Autodesk Fusion 360 part; units mm, degrees
(part 5 of 6)
extrude "Extrude1" add sketch "Back Panel Support Left " along normal blind 21
equation "d1 = 323 mm - 21 mm - 32 mm"

design "9V Battery Compartment"
Autodesk Fusion 360 part; units mm, degrees
sketch "Battery Body" plane through (0, 0, 0) normal (0, 0, 1) x (1, 0, 0)
  line L0 (0, 0) -> (24, 0)
  line L1 (24, 0) -> (24, 16)
  line L2 (24, 16) -> (0, 16)
  line L3 (0, 16) -> (0, 0)
  dimension "d1" = 24
  dimension "d2" = 16
  constraint horizontal L0
  constraint vertical L1
  constraint horizontal L2
  constraint vertical L3
  constraint coincident L0.start L3.end
  measures "d1" distance of L0.start L0.end
  measures "d2" distance of L0.end L1.end
extrude "Extrude1" add sketch "Battery Body" along normal blind 26 makes body 1
extrude "Extrude2" add 1 faces at (8, 10.6667, 26) along direction (0, 0, 1) blind 3 separate body on bodies 1 makes body 2
extrude "Extrude3" add 1 faces at (8, 10.6667, 29) along direction (0, 0, 1) blind 0.5 separate body on bodies 2 makes body 3
extrude "Extrude4" add 1 faces at (8, 10.6667, 29.5) along direction (0, 0, 1) blind 13.5 separate body on bodies 3 makes body 4
fillet "Fillet1" radius 1 16 edges at (0, 0, 13) (24, 0, 13) (24, 16, 13) (0, 16, 13) (0, 0, 27.5) (24, 0, 27.5) (24, 16, 27.5) (0, 16, 27.5) (0, 0, 29.25) (24, 0, 29.25) (24, 16, 29.25) (0, 16, 29.25) (0, 0, 36.25) (24, 0, 36.25) (24, 16, 36.25) (0, 16, 36.25) on bodies 1 2 3 4
sketch "Battery Terminals" plane through (0, 0, 43) normal (0, 0, 1) x (-1, 0, 0)
  arc A0 (-1, -16) -> (0, -15) centre (-1, -15) ccw
  line L0 (0, -15) -> (0, -1)
  arc A1 (0, -1) -> (-1, 0) centre (-1, -1) ccw
  line L1 (-1, 0) -> (-23, 0)
  arc A2 (-23, 0) -> (-24, -1) centre (-23, -1) ccw
  line L2 (-24, -1) -> (-24, -15)
  arc A3 (-24, -15) -> (-23, -16) centre (-23, -15) ccw
  line L3 (-23, -16) -> (-1, -16)
  circle A4 centre (-6, -8) radius 3
  circle A5 centre (-18, -8) radius 2
  circle A6 centre (-18, -8) radius 3
  circle A7 centre (-6, -8) radius 4
  dimension "d13" = 4
  dimension "d14" = 6
  dimension "d15" = 6
  dimension "d16" = 8
  dimension "d17" = 8
  dimension "d18" = 8
  dimension "d19" = 6
  dimension "d20" = 6
  constraint concentric A5 A6
  constraint concentric A4 A7
  measures "d13" diameter of A5
  measures "d14" diameter of A6
  measures "d15" diameter of A4
  measures "d16" diameter of A7
  measures "d17" distance of L1 A5.centre
  measures "d18" distance of L1 A4.centre
  measures "d19" distance of L0 A4.centre
  measures "d20" distance of L2 A5.centre
extrude "Extrude5" add sketch "Battery Terminals" along normal blind 4 separate body contours A6 | A7 makes body 5 at (15.0149, 8.2987, 44.3333) makes body 6 at (2.0199, 8.3983, 44.3333)
sketch "Battery Compartment" plane through (0, 0, 0) normal (0, 1, 0) x (1, 0, 0)
  line L0 (40, 0) -> (70, 0)
  line L1 (70, 0) -> (70, -53)
  line L2 (70, -53) -> (40, -53)
  line L3 (40, -53) -> (40, 0)
  dimension "d25" = 30
  dimension "d26" = 53
  constraint horizontal L0
  constraint vertical L1
  constraint horizontal L2
  constraint vertical L3
  measures "d25" distance of L0.start L0.end
  measures "d26" distance of L0.end L1.end
extrude "Extrude1'" add sketch "Battery Compartment" against normal blind 2 separate body makes body 7 in component "9V Battey Compartment"
sketch "Battery Compartment Fins" plane through (0, -2, 0) normal (0, -1, 0) x (1, 0, 0)
  line L0 (70, 53) -> (40, 53)
  line L1 (40, 53) -> (40, 0)
  line L2 (40, 0) -> (70, 0)
  line L3 (70, 0) -> (70, 53)
  line L4 (40, 53) -> (41, 53)
  line L5 (41, 53) -> (41, 24)
  line L6 (41, 24) -> (40, 24)
  line L7 (40, 24) -> (40, 53)
  line L8 (41, 53) -> (70, 53)
  line L9 (70, 53) -> (70, 52)
  line L10 (70, 52) -> (41, 52)
  line L11 (41, 52) -> (41, 53)
  line L12 (70, 52) -> (69, 52)
  line L13 (69, 52) -> (69, 24)
  line L14 (69, 24) -> (70, 24)
  line L15 (70, 24) -> (70, 52)
  line L16 (45, 0) -> (65, 0)
  line L17 (65, 0) -> (65, 3)
  line L18 (65, 3) -> (45, 3)
  line L19 (45, 3) -> (45, 0)
  dimension "d29" = 1
  dimension "d30" = 1
  dimension "d31" = 1
  dimension "d32" = 28
  dimension "d33" = 3
  dimension "d34" = 20
  dimension "d35" = 5
  constraint horizontal L4
  constraint vertical L5
  constraint horizontal L6
  constraint vertical L7
  constraint coincident L0.end L1.start
  constraint horizontal L8
  constraint vertical L9
  constraint horizontal L10
  constraint vertical L11
  constraint coincident L3 L9.end
  constraint horizontal L12
  constraint vertical L13
  constraint horizontal L14
  constraint vertical L15
  constraint collinear L6 L14
  constraint horizontal L16
  constraint vertical L17
  constraint horizontal L18
  constraint vertical L19
  constraint coincident L2 L16.start
  measures "d29" distance of L5.end L6.end
  measures "d30" distance of L13 L15
  measures "d31" distance of L8 L10
  measures "d32" distance of L9.end L14.end
  measures "d33" distance of L16.end L17.end
  measures "d34" distance of L16.start L16.end
  measures "d35" distance of L1 L19
extrude "Extrude2'" add sketch "Battery Compartment Fins" along normal blind 16 contours L0 L3 L5 L8 L9 L10 L11 L12 | L0 L1 L4 L5 L6 L7 L11 | L3 L10 L12 L13 L14 L15 bodies 7 in component "9V Battey Compartment"
chamfer "Chamfer1" distance 28 distance2 16 2 edges at (69.5, -18, 24) (40.5, -18, 24) measured on face at (50.3333, -18, 52.6667) measured on face at (50.3333, -18, 52.6667) on bodies 7 in component "9V Battey Compartment"
extrude "Extrude3'" add sketch "Battery Compartment Fins" along normal blind 11 contours L2 L16 L17 L18 L19 bodies 7 in component "9V Battey Compartment"
chamfer "Chamfer2" distance 2 distance2 11 1 edges at (55, -13, 0) measured on face at (58.3333, -13, 1) on bodies 7 in component "9V Battey Compartment"
sketch "Compartment Terminals" plane through (0, 0, 52) normal (0, 0, -1) x (1, 0, 0)
  line L0 (41, 2) -> (69, 2)
  line L1 (69, 2) -> (69, 18)
  line L2 (69, 18) -> (41, 18)
  line L3 (41, 18) -> (41, 2)
  circle A0 centre (49, 10) radius 3
  circle A1 centre (61, 10) radius 4
  circle A2 centre (61, 10) radius 3
  circle A3 centre (49, 10) radius 2
  line L4 (70, 2) -> (41, 2)
  dimension "d44" = 12
  dimension "d45" = 6
  dimension "d46" = 8
  dimension "d47" = 4
  dimension "d48" = 6
  dimension "d49" = 8
  dimension "d51" = 8
  dimension "d52" = 8
  constraint concentric A1 A2
  constraint concentric A0 A3
  measures "d44" distance of A0.centre A1.centre
  measures "d45" diameter of A2
  measures "d46" diameter of A1
  measures "d47" diameter of A3
  measures "d48" diameter of A0
  measures "d49" distance of A0.centre L4
  measures "d51" distance of A1.centre L4
  measures "d52" distance of L3 A0.centre
extrude "Extrude6" add sketch "Compartment Terminals" along normal blind 4 separate body contours A0 | A1 makes body 8 at (51.9851, -9.7013, 50.6667) makes body 9 at (64.9801, -9.6017, 50.6667)
fillet "Fillet3" radius 0.5 4 edges at (46.203, -8.9152, 48) (47.1353, -10.7232, 48) (58.203, -11.0848, 48) (57.2707, -8.5535, 48) on bodies 8 9
copy_body "CutPasteBodies1" bodies 9 removing the originals makes body 10 in component "9V Battey Compartment"
copy_body "CutPasteBodies2" bodies 8 removing the originals makes body 11 in component "9V Battey Compartment"
copy_body "Body->Comp1" bodies 1 removing the originals makes body 12 in component "9V Battery"
copy_body "CutPasteBodies1'" bodies 2 removing the originals makes body 13 in component "9V Battery"
copy_body "CutPasteBodies2'" bodies 3 removing the originals makes body 14 in component "9V Battery"
copy_body "CutPasteBodies3" bodies 4 removing the originals makes body 15 in component "9V Battery"
copy_body "CutPasteBodies4" bodies 5 removing the originals makes body 16 in component "9V Battery"
copy_body "CutPasteBodies5" bodies 6 removing the originals makes body 17 in component "9V Battery"
fillet "Fillet1'" radius 0.5 4 edges at (20.797, 9.0848, 47) (19.8647, 7.2768, 47) (8.797, 6.9152, 47) (9.7293, 9.4465, 47) on bodies 16 17 in component "9V Battery"
sketch "Compartment Bottom Fin Round Part" plane through (25, 0, 0) normal (1, 0, 0) x (0, 1, 0)
  line L0 (-11, 2) -> (0, 0)
  line L1 (0, 0) -> (0, 3)
  line L2 (0, 3) -> (-11, 3)
  line L3 (-11, 3) -> (-11, 2)
  ellipse E0 centre (-9, 3) end of major axis (-9, 2.5) minor radius 2
  line L4 (-9, 3.5) -> (-9, 2.5) construction
  line L5 (-11, 3) -> (-7, 3) construction
  dimension "d66" = 4
  dimension "d67" = 2
  constraint coincident L2 E0.centre
  constraint perpendicular L2 L4
  constraint coincident E0 L4.start
  constraint coincident E0 L4.end
  constraint coincident E0 L2.end
  constraint coincident E0 L5.end
  measures "d67" distance of L2.end E0.centre
extrude "Extrude4'" add sketch "Compartment Bottom Fin Round Part" against normal blind 20 contours L2 E0 picked at (-9.0518, 3.1662) sketch seen with x (1, 0, 0) y (0, 1, 0) z (0, 0, 1) at (40, -2, 0) bodies 7 in component "9V Battey Compartment"
combine "Combine1" operation add target body 12 tool bodies 13 14 in component "9V Battery"
component "9V Battey Compartment" placed x (1, 0, 0) y (0, 1, 0) z (0, 0, 1) at (-40, 2, 0)
component "9V Battery" placed x (1, 0, 0) y (0, 1, 0) z (0, 0, 1) at (3, -16, 5)

design "Savöx SH 0255 MG Micro Servo"
Autodesk Fusion 360 part; units mm, degrees
sketch "Servo Side Profile" plane through (0, 0, 0) normal (1, 0, 0) x (0, 1, 0)
  line L0 (0, 0) -> (22, 0)
  line L1 (22, 0) -> (22, 16)
  line L2 (22, 16) -> (27, 16)
  line L3 (27, 16) -> (27, 18)
  line L4 (27, 18) -> (22, 18)
  line L5 (22, 18) -> (22, 22)
  line L6 (22, 22) -> (0, 22)
  line L7 (0, 22) -> (0, 18)
  line L8 (0, 18) -> (-5, 18)
  line L9 (-5, 18) -> (-5, 16)
  line L10 (-5, 16) -> (0, 16)
  line L11 (0, 16) -> (0, 0)
  dimension "d1" = 22
  dimension "d2" = 22
  dimension "d3" = 16
  dimension "d4" = 16
  dimension "d5" = 2
  dimension "d6" = 2
  dimension "d7" = 4
  dimension "d9" = 5
  dimension "d10" = 5
  constraint coincident L0.start L11.end
  constraint horizontal L0
  constraint perpendicular L0 L1
  constraint perpendicular L1 L2
  constraint perpendicular L2 L3
  constraint perpendicular L3 L4
  constraint perpendicular L4 L5
  constraint perpendicular L3 L6
  constraint perpendicular L6 L7
  constraint perpendicular L3 L8
  constraint perpendicular L8 L9
  constraint perpendicular L9 L10
  constraint perpendicular L0 L11
  constraint collinear L7 L11
  measures "d1" distance of L0.start L0.end
  measures "d2" distance of L5.end L6.end
  measures "d3" distance of L0.end L1.end
  measures "d4" distance of L10.end L0.start
  measures "d5" distance of L2.end L3.end
  measures "d6" distance of L8.end L9.end
  measures "d7" distance of L6.end L7.end
  measures "d9" distance of L3.end L4.end
  measures "d10" distance of L7.end L8.end
extrude "Extrude1" add sketch "Servo Side Profile" along normal blind 11 makes body 1
sketch "Top Cylinders" plane through (0, 0, 22) normal (0, 0, 1) x (-1, 0, 0)
  line L0 (0, -22) -> (0, 0)
  line L1 (0, 0) -> (-11, 0)
  line L2 (-11, 0) -> (-11, -22)
  line L3 (-11, -22) -> (0, -22)
  circle A0 centre (-5.5, -5.5) radius 5.5
  circle A1 centre (-5.5, -11) radius 2.5
  dimension "d13" = 5.5
  dimension "d14" = 5.5
  dimension "d15" = 11
  dimension "d16" = 5.5
  dimension "d17" = 11
  dimension "d18" = 5
  measures "d13" distance of L2 A0.centre
  measures "d14" distance of L1 A0.centre
  measures "d15" diameter of A0
  measures "d16" distance of L2 A1.centre
  measures "d17" distance of L1 A1.centre
  measures "d18" diameter of A1
extrude "Extrude2" add sketch "Top Cylinders" along normal blind 5 contours A0 A1 | A0 A1 | A0 A1 bodies 1
sketch "Turning Gear" plane through (0, 0, 27) normal (0, 0, 1) x (-1, 0, 0)
  arc A0 (-7.9346, -10.4318) -> (-3.0654, -10.4318) centre (-5.5, -11) ccw
  arc A1 (-3.0654, -10.4318) -> (-7.9346, -10.4318) centre (-5.5, -5.5) ccw
  circle A2 centre (-5.5, -5.5) radius 2.5
  dimension "d21" = 5
  constraint concentric A1 A2
  measures "d21" diameter of A2
extrude "Extrude3" add sketch "Turning Gear" along normal blind 3 separate body contours A2 makes body 2
equation "d13 = ( 11 / 2 ) * 1 mm"
equation "d14 = ( 11 / 2 ) * 1 mm"
equation "d16 = ( 11 / 2 ) * 1 mm"
equation "d17 = ( 22 / 2 ) * 1 mm"

design "Colour Detection Mechanism Top Panel Placeholder"
Autodesk Fusion 360 part; units mm, degrees
sketch "Sorting Mechanism Top Panel Placeholder" plane through (0, 0, 0) normal (0, 0, 1) x (1, 0, 0)
  line L0 (0, 0) -> (28, 0)
  line L1 (28, 0) -> (28, 10)
  line L2 (28, 10) -> (0, 10)
  line L3 (0, 10) -> (0, 0)
  dimension "d1" = 10
  dimension "d2" = 28
  constraint horizontal L0
  constraint vertical L1
  constraint horizontal L2
  constraint vertical L3
  constraint coincident L0.start L3.end
  measures "d1" distance of L0.end L1.end
  measures "d2" distance of L0.start L0.end
extrude "Extrude1" add sketch "Sorting Mechanism Top Panel Placeholder" along normal blind 12

design "Unsorted Smarties Top Panel"
Autodesk Fusion 360 part; units mm, degrees
sketch "Unsorted Smarties Top" plane through (0, 0, 0) normal (0, 0, 1) x (1, 0, 0)
  line L0 (0, 0) -> (270, 0)
  line L1 (270, 0) -> (270, 48)
  line L2 (270, 48) -> (0, 48)
  line L3 (0, 48) -> (0, 0)
  dimension "d1" = 270
  dimension "d2" = 48
  constraint horizontal L0
  constraint vertical L1
  constraint horizontal L2
  constraint vertical L3
  constraint coincident L0.start L3.end
  measures "d1" distance of L0.start L0.end
  measures "d2" distance of L0.end L1.end
extrude "Extrude1" add sketch "Unsorted Smarties Top" along normal blind 6
sketch "Sketch2" plane through (0, 0, 0) normal (0, 0, -1) x (1, 0, 0)
  line L0 (0, 0) -> (0, -48)
  line L1 (0, -48) -> (270, -48)
  line L2 (270, -48) -> (270, 0)
  line L3 (270, 0) -> (0, 0)
  line L4 (5, -10) -> (265, -10)
  line L5 (265, -10) -> (265, -20)
  line L6 (265, -20) -> (5, -20)
  line L7 (5, -20) -> (5, -10)
  line L8 (5, -29) -> (265, -29)
  line L9 (265, -29) -> (265, -39)
  line L10 (265, -39) -> (5, -39)
  line L11 (5, -39) -> (5, -29)
  dimension "d6" = 5
  dimension "d7" = 5
  dimension "d8" = 5
  dimension "d9" = 5
  dimension "d10" = 10
  dimension "d11" = 10
  dimension "d12" = 9
  dimension "d13" = 10
  constraint horizontal L4
  constraint vertical L5
  constraint horizontal L6
  constraint vertical L7
  constraint horizontal L8
  constraint vertical L9
  constraint horizontal L10
  constraint vertical L11
  measures "d6" distance of L2 L5
  measures "d7" distance of L2 L9
  measures "d8" distance of L0 L7
  measures "d9" distance of L0 L11
  measures "d10" distance of L4.start L6.end
  measures "d11" distance of L3 L4
  measures "d12" distance of L6 L8
  measures "d13" distance of L8.start L10.end
extrude "Extrude2" cut sketch "Sketch2" against normal blind 4 contours L4 L5 L6 L7 | L8 L9 L10 L11
sketch "Sketch3" plane through (0, 0, 4) normal (0, 0, -1) x (1, 0, 0)
  line L0 (5, -20) -> (265, -20)
  line L1 (265, -20) -> (265, -10)
  line L2 (265, -10) -> (5, -10)
  line L3 (5, -10) -> (5, -20)
  line L4 (265, -10) -> (255, -10)
  line L5 (255, -10) -> (255, -20)
  line L6 (255, -20) -> (265, -20)
  line L7 (265, -20) -> (265, -10)
  line L8 (265, -29) -> (255, -29)
  line L9 (255, -29) -> (255, -39)
  line L10 (255, -39) -> (265, -39)
  line L11 (265, -39) -> (265, -29)
  constraint horizontal L4
  constraint vertical L5
  constraint horizontal L6
  constraint vertical L7
  constraint coincident L0 L5.end
  constraint coincident L1.end L2.start
  constraint horizontal L8
  constraint vertical L9
  constraint horizontal L10
  constraint vertical L11
extrude "Extrude3" cut sketch "Sketch3" against normal blind 2 contours L0 L1 L2 L4 L5 L6 L7 | L8 L9 L10 L11
equation "mdfThickness = 6 mm"
equation "d4 = mdfThickness"

design "Control Panel Front"
Autodesk Fusion 360 part; units mm, degrees
sketch "Control Panel Front" plane through (0, 0, 0) normal (0, 1, 0) x (1, 0, 0)
  line L0 (0, 0) -> (270, 0)
  line L1 (270, 0) -> (270, -43)
  line L2 (270, -43) -> (0, -43)
  line L3 (0, -43) -> (0, 0)
  dimension "d6" = 270
  dimension "d7" = 43
  constraint horizontal L0
  constraint vertical L1
  constraint horizontal L2
  constraint vertical L3
  constraint coincident L0.start L3.end
  measures "d6" distance of L0.start L0.end
  measures "d7" distance of L0.end L1.end
extrude "Extrude1" add sketch "Control Panel Front" along normal blind 6
equation "MDFThickness = 6 mm"
equation "d2 = MDFThickness"
equation "d7 = sidePanelControlPanelHeight - 2 * sidePanelClearance - 2 * MDFThickness"
equation "sidePanelClearance = 10 mm"
equation "sidePanelControlPanelHeight = 75 mm"

design "Name Sign LED Holder"
Autodesk Fusion 360 part; units mm, degrees
sketch "Sketch1" plane through (0, 0, 0) normal (0, 1, 0) x (1, 0, 0)
  line L0 (2.4744, -68.9852) -> (7.4744, -68.9852)
  line L1 (7.4744, -68.9852) -> (7.4744, -22.3387)
  line L2 (7.4744, -22.3387) -> (36.754, -10.3303)
  line L3 (36.754, -10.3303) -> (34.8567, -5.7042)
  line L4 (34.8567, -5.7042) -> (2.4744, -18.9852)
  line L5 (2.4744, -18.9852) -> (2.4744, -68.9852)
  line L6 (2.4744, -68.9852) -> (7.4744, -66.9345)
  line L7 (34.8567, -5.7042) -> (34.8567, -11.1084)
  dimension "d1" = 5
  dimension "d2" = 5
  dimension "d3" = 112.3
  dimension "d16" = 50
  dimension "d18" = 22.3
  dimension "d20" = 35
  constraint horizontal L0
  constraint perpendicular L0 L1
  constraint perpendicular L2 L3
  constraint perpendicular L0 L5
  constraint parallel L2 L4
  constraint coincident L1 L6.end
  constraint parallel L2 L6
  constraint coincident L2 L7.end
  constraint vertical L7
  measures "d1" distance of L0.start L0.end
  measures "d2" distance of L2.end L3.end
  measures "d3" angle of L1 L2
  measures "d16" distance of L0.start L4.end
  measures "d18" angle of L0 L6
  measures "d20" distance of L3.end L4.end
extrude "Extrude1" add sketch "Sketch1" along normal blind 220 contours L1 L2 L4 L5 L6 L7
sketch "Sketch2" plane through (2.4744, 0, 0) normal (-1, 0, 0) x (0, -1, 0)
  line L0 (0, 18.9852) -> (0, 68.9852)
  line L1 (-220, 68.9852) -> (-220, 18.9852)
  line L2 (-220, 18.9852) -> (0, 18.9852)
  line L3 (-215, 66.9852) -> (-5, 66.9852)
  line L4 (-5, 66.9852) -> (-5, 56.9852)
  line L5 (-5, 56.9852) -> (-215, 56.9852)
  line L6 (-215, 56.9852) -> (-215, 66.9852)
  line L7 (-215, 52.9852) -> (-5, 52.9852)
  line L8 (-5, 52.9852) -> (-5, 42.9852)
  line L9 (-5, 42.9852) -> (-215, 42.9852)
  line L10 (-215, 42.9852) -> (-215, 52.9852)
  line L11 (-5, 66.9852) -> (-15, 66.9852)
  line L12 (-15, 56.9852) -> (-5, 56.9852)
  line L13 (-5, 56.9852) -> (-5, 66.9852)
  line L14 (-5, 52.9852) -> (-15, 52.9852)
  line L15 (-15, 42.9852) -> (-5, 42.9852)
  line L16 (-5, 42.9852) -> (-5, 52.9852)
  line L17 (0, 68.9852) -> (-220, 68.9852)
  dimension "d6" = 210
  dimension "d7" = 210
  dimension "d8" = 5
  dimension "d9" = 5
  dimension "d12" = 10
  dimension "d13" = 10
  dimension "d22" = 4
  dimension "d30" = 2
  constraint horizontal L3
  constraint vertical L4
  constraint horizontal L5
  constraint vertical L6
  constraint horizontal L7
  constraint vertical L8
  constraint horizontal L9
  constraint vertical L10
  constraint horizontal L11
  constraint horizontal L12
  constraint vertical L13
  constraint coincident L5 L12.start
  constraint horizontal L14
  constraint horizontal L15
  constraint vertical L16
  constraint coincident L9 L15.start
  measures "d6" distance of L3.start L3.end
  measures "d7" distance of L8.end L9.end
  measures "d8" distance of L1 L6
  measures "d9" distance of L0 L8
  measures "d12" distance of L3.start L5.end
  measures "d13" distance of L7.start L9.end
  measures "d22" distance of L5 L7
  measures "d30" distance of L3 L17
extrude "Extrude2" cut sketch "Sketch2" against normal blind 3 contours L3 L4 L5 L6 L11 L12 L13 | L7 L8 L9 L10 L14 L15 L16
sketch "Sketch3" plane through (5.4744, 0, 0) normal (-1, 0, 0) x (0, -1, 0)
  line L0 (-215, 56.9852) -> (-5, 56.9852)
  line L1 (-5, 56.9852) -> (-5, 66.9852)
  line L2 (-5, 66.9852) -> (-215, 66.9852)
  line L3 (-215, 66.9852) -> (-215, 56.9852)
  line L4 (-5, 66.9852) -> (-15, 66.9852)
  line L5 (-15, 66.9852) -> (-15, 56.9852)
  line L6 (-15, 56.9852) -> (-5, 56.9852)
  line L7 (-5, 56.9852) -> (-5, 66.9852)
  dimension "d33" = 10
  dimension "d34" = 10
  constraint horizontal L4
  constraint vertical L5
  constraint horizontal L6
  constraint vertical L7
  constraint coincident L0 L5.end
  constraint coincident L1.end L2.start
  measures "d33" distance of L1.end L4.end
  measures "d34" distance of L1.end L0.end
sketch "Sketch4" plane through (5.4744, 0, 0) normal (-1, 0, 0) x (0, -1, 0)
  line L0 (-215, 42.9852) -> (-5, 42.9852)
  line L1 (-5, 42.9852) -> (-5, 52.9852)
  line L2 (-215, 52.9852) -> (-215, 42.9852)
  line L3 (-5, 52.9852) -> (-15, 52.9852)
  line L4 (-15, 52.9852) -> (-15, 42.9852)
  line L5 (-15, 42.9852) -> (-5, 42.9852)
  line L6 (-5, 42.9852) -> (-5, 52.9852)
  line L7 (-5, 52.9852) -> (-215, 52.9852)
  dimension "d26" = 10
  dimension "d27" = 10
  constraint horizontal L3
  constraint vertical L4
  constraint horizontal L5
  constraint vertical L6
  constraint coincident L0 L4.end
  constraint coincident L1.end L3.start
  measures "d26" distance of L1.end L3.end
  measures "d27" distance of L1.end L0.end
extrude "Extrude3" cut sketch "Sketch3" sketch "Sketch4" against normal blind 2 contours L0 L1 L2 L4 L5 L6 L7 of sketch 2 contours L0 L1 L3 L4 L5 L6 L7
equation "d4 = 200 mm + 10 mm + 5 mm + 5 mm"
equation "d6 = 200 mm + 10 mm"
equation "d7 = 200 mm + 10 mm"

design "Smartie Hopper"
Autodesk Fusion 360 part; units mm, degrees
sketch "Bottom opening" plane through (0, 0, 0) normal (0, 0, 1) x (1, 0, 0)
  line L0 (0, 0) -> (18, 0)
  line L1 (18, 0) -> (18, 18)
  line L2 (18, 18) -> (0, 18)
  line L3 (0, 18) -> (0, 0)
  line L4 (-4, 22) -> (22, 22)
  line L5 (22, 22) -> (22, -4)
  line L6 (22, -4) -> (-4, -4)
  line L7 (-4, -4) -> (-4, 22)
  dimension "d3" = 18
  dimension "d4" = 18
  dimension "d5" = 4
  dimension "d6" = 4
  dimension "d7" = 4
  dimension "d8" = 4
  constraint horizontal L0
  constraint vertical L1
  constraint horizontal L2
  constraint vertical L3
  constraint coincident L0.start L3.end
  constraint horizontal L4
  constraint vertical L5
  constraint horizontal L6
  constraint vertical L7
  measures "d3" distance of L0.start L0.end
  measures "d4" distance of L0.end L1.end
  measures "d5" distance of L2 L4
  measures "d6" distance of L0 L6
  measures "d7" distance of L1 L5
  measures "d8" distance of L3 L7
ref_plane "WorkPlane1" through (0, 0, 34) normal (0, 0, 1) x (1, 0, 0)
sketch "Top opening" plane through (0, 0, 34) normal (0, 0, 1) x (1, 0, 0)
  line L0 (18, 18) -> (0, 18)
  line L1 (18, 0) -> (18, 18)
  line L2 (0, 0) -> (18, 0)
  line L3 (0, 18) -> (0, 0)
  line L4 (-4, 22) -> (22, 22)
  line L5 (22, -4) -> (-4, -4)
  line L6 (22, 22) -> (22, -4)
  line L7 (-4, -4) -> (-4, 22)
  line L8 (-36, 44) -> (54, 44)
  line L9 (54, 44) -> (54, -26)
  line L10 (54, -26) -> (-36, -26)
  line L11 (-36, -26) -> (-36, 44)
  line L12 (-39, 47) -> (57, 47)
  line L13 (57, 47) -> (57, -29)
  line L14 (57, -29) -> (-39, -29)
  line L15 (-39, -29) -> (-39, 47)
  line L16 (-40, 48) -> (58, 48)
  line L17 (58, 48) -> (58, -30)
  line L18 (58, -30) -> (-40, -30)
  line L19 (-40, -30) -> (-40, 48)
  dimension "d14" = 3
  dimension "d15" = 4
  dimension "d16" = 3
  dimension "d17" = 4
  dimension "d18" = 90
  dimension "d19" = 70
  dimension "d20" = 3
  dimension "d21" = 4
  dimension "d22" = 3
  dimension "d23" = 4
  dimension "d24" = 32
  dimension "d25" = 32
  dimension "d26" = 22
  dimension "d27" = 22
  constraint horizontal L8
  constraint vertical L9
  constraint horizontal L10
  constraint vertical L11
  constraint horizontal L12
  constraint vertical L13
  constraint horizontal L14
  constraint vertical L15
  constraint horizontal L16
  constraint vertical L17
  constraint horizontal L18
  constraint vertical L19
  measures "d14" distance of L9 L13
  measures "d15" distance of L9 L17
  measures "d16" distance of L11 L15
  measures "d17" distance of L11 L19
  measures "d18" distance of L8.start L8.end
  measures "d19" distance of L8.end L9.end
  measures "d20" distance of L8 L12
  measures "d21" distance of L8 L16
  measures "d22" distance of L10 L14
  measures "d23" distance of L10 L18
  measures "d24" distance of L7 L11
  measures "d25" distance of L6 L9
  measures "d26" distance of L4 L8
  measures "d27" distance of L5 L10
loft "Loft1" add profiles "Top opening", "Bottom opening" section 1 contours L8 L9 L10 L11 | L12 L13 L14 L15 | L16 L17 L18 L19 section 2 contours L0 L1 L2 L3 | L4 L5 L6 L7
extrude "Extrude1" cut sketch "Top opening" against normal blind 6 contours L16 L17 L18 L19
extrude "Extrude4" add 1 faces at (25, -3.6667, 34) along direction (0, 0, -1) blind 6
sketch "Support lip" plane through (57, 0, 0) normal (1, 0, 0) x (0, 1, 0)
  line L0 (47, 28) -> (47, 34)
  line L1 (47, 34) -> (-29, 34)
  line L2 (-29, 34) -> (-29, 28)
  line L3 (-29, 28) -> (77, 28)
  line L4 (77, 28) -> (77, 23)
  line L5 (77, 23) -> (-29, 23)
  line L6 (-29, 23) -> (-29, 28)
  line L7 (-29, 28) -> (47, 28)
  line L8 (-29, 28) -> (9, 28)
  line L9 (9, 28) -> (9, 23)
  line L10 (9, 23) -> (-29, 23)
  line L11 (-29, 23) -> (-29, 28)
  dimension "d31" = 6
  dimension "d34" = 5
  dimension "d35" = 30
  dimension "d50" = 38
  constraint horizontal L3
  constraint vertical L4
  constraint horizontal L5
  constraint vertical L6
  constraint collinear L2 L6
  constraint horizontal L8
  constraint vertical L9
  constraint horizontal L10
  constraint vertical L11
  constraint coincident L5 L9.end
  constraint coincident L2.end L3.start
  measures "d31" distance of L1 L3
  measures "d34" distance of L2.end L5.end
  measures "d35" distance of L0.end L3.end
  measures "d50" distance of L9 L11
extrude "Extrude2" add sketch "Support lip" along normal blind 30 and the other way blind 126 contours L3 L5 L6 L7 L8 L9 L10 L11
extrude "Extrude5" add sketch "Support lip" against normal blind 78 from surface at -48 contours L3 L4 L5 L7 L9
fillet "Fillet4" radius 5 5 edges at (87, 9, 25.5) (87, -29, 25.5) (9, 77, 25.5) (-69, 77, 25.5) (-69, -29, 25.5)
loft "Loft2" cut profiles "Top opening", "Bottom opening" section 1 contours L8 L9 L10 L11 section 2 contours L0 L1 L2 L3
fillet "Fillet3" radius 12.803 4 edges at (-18, 31, 17) (-18, -13, 17) (36, -13, 17) (36, 31, 17)
fillet "Fillet5" radius 18.495 4 edges at (-16.1765, -12.7941, 11.5) (-16.1765, 30.7941, 11.5) (36.8235, 32.7059, 14) (34.1765, -12.7941, 11.5)
equation "bottom_outlet_size = 18 mm"
equation "hopper_wall_thickness = 4 mm"
equation "d3 = bottom_outlet_size"
equation "d4 = bottom_outlet_size"
equation "d5 = hopper_wall_thickness"
equation "d6 = hopper_wall_thickness"
equation "d7 = hopper_wall_thickness"
equation "d8 = hopper_wall_thickness"
equation "hopper_height = 34 mm"
equation "d10 = hopper_height"
equation "acrylic_thickness = 3 mm"
equation "top_outlet_width = 90 mm"
equation "top_outlet_depth = 70 mm"
equation "d14 = acrylic_thickness"
equation "d15 = hopper_wall_thickness"
equation "d16 = acrylic_thickness"
equation "d17 = hopper_wall_thickness"
equation "d18 = top_outlet_width"
equation "d19 = top_outlet_depth"
equation "d20 = acrylic_thickness"
equation "d21 = hopper_wall_thickness"
equation "d22 = acrylic_thickness"
equation "d23 = hopper_wall_thickness"
equation "d24 = ( top_outlet_width - ( bottom_outlet_size + 2 * hopper_wall_thickness ) ) / 2"
equation "d26 = ( top_outlet_depth - ( bottom_outlet_size + 2 * hopper_wall_thickness ) ) / 2"
equation "MDF_thickness = 6 mm"
equation "d31 = MDF_thickness"
equation "support_lip_width = 30 mm"
equation "support_lip_thickness = 5 mm"
equation "d34 = support_lip_thickness"
equation "d35 = support_lip_width"
equation "d36 = support_lip_width"
equation "d38 = ( top_outlet_width + 2 * acrylic_thickness ) + support_lip_width"
equation "d50 = ( top_outlet_depth / 2 ) + acrylic_thickness"
equation "d51 = -( top_outlet_width / 2 ) - acrylic_thickness"
equation "d52 = -( top_outlet_width / 2 ) - acrylic_thickness - support_lip_width"

design "1.5 Volt Label"
Autodesk Fusion 360 part; units mm, degrees
sketch "Sticker" plane through (0, 0, 0) normal (0, 1, 0) x (1, 0, 0)
  line L0 (0, 0) -> (35, 0)
  line L1 (35, 0) -> (35, -12)
  line L2 (35, -12) -> (0, -12)
  line L3 (0, -12) -> (0, 0)
  dimension "d1" = 35
  dimension "d2" = 12
  constraint horizontal L0
  constraint vertical L1
  constraint horizontal L2
  constraint vertical L3
  constraint coincident L0.start L3.end
  measures "d1" distance of L0.start L0.end
  measures "d2" distance of L0.end L1.end
extrude "Extrude1" add sketch "Sticker" along normal blind 0.01 makes body 1
sketch "Text" plane through (0, 0, 0) normal (0, -1, 0) x (1, 0, 0)
  line L0 (35, 12) -> (0, 12)
  line L1 (0, 12) -> (0, 0)
  line L2 (0, 0) -> (35, 0)
  line L3 (35, 0) -> (35, 12)
  line L4 (0, 0) -> (35, 0) construction
  line L5 (35, 0) -> (35, 12) construction
  line L6 (35, 12) -> (0, 12) construction
  line L7 (0, 12) -> (0, 0) construction
  dimension "d5" = 5
  text T0 "2 × 1.5 V" font "Arial" height 5 align centre middle in box 35 x 12 at (0, 0) x (1, 0) y (0, 1) spacing 1 kerned
  constraint coincident L2.end
  constraint coincident L0.end
extrude "Extrude2" add sketch "Text" along normal blind 0.01 separate body text T0 makes body 2 at (10.575, 0, 6.465) makes body 3 at (27.7817, 0, 7.2892) makes body 4 at (22.8908, 0, 8.2362) makes body 5 at (20.1748, 0, 3.7331) makes body 6 at (17.5872, 0, 6.4775) makes body 7 at (4.9417, 0, 3.6967)

design "Base Plate Support"
Autodesk Fusion 360 part; units mm, degrees
sketch "Control Panel Support" plane through (0, 0, 0) normal (1, 0, 0) x (0, 1, 0)
  line L0 (0, 0) -> (48, 0)
  line L1 (48, 0) -> (48, 50)
  line L2 (48, 50) -> (0, 50)
  line L3 (0, 50) -> (0, 0)
  dimension "d1" = 48
  dimension "d2" = 50
  constraint horizontal L0
  constraint vertical L1
  constraint horizontal L2
  constraint vertical L3
  constraint coincident L0.start L3.end
  measures "d1" distance of L0.start L0.end
  measures "d2" distance of L0.end L1.end
extrude "Extrude1" add sketch "Control Panel Support" along normal blind 12
equation "pineThickness = 12 mm"
equation "d4 = pineThickness"
equation "mdfThickness = 6 mm"

design "Back Panel"
Autodesk Fusion 360 part; units mm, degrees
sketch "Back Panel" plane through (0, 0, 0) normal (1, 0, 0) x (0, 1, 0)
  line L0 (0, 0) -> (6, 0)
  line L1 (6, 0) -> (6, 500.8)
  line L2 (0, 500.8) -> (0, 0)
  line L3 (0, 500.8) -> (0, 503.263)
  line L4 (6, 500.8) -> (0, 503.263)
  dimension "d8" = 6
  dimension "d9" = 500.8
  dimension "d10" = 2.463
  dimension "d11" = 112.318
  constraint horizontal L0
  constraint vertical L1
  constraint vertical L2
  constraint coincident L0.start L2.end
  measures "d8" distance of L0.start L0.end
  measures "d9" distance of L0.end L1.end
  measures "d10" distance of L2.start L3.end
  measures "d11" angle of L1 L4
extrude "Extrude2" add sketch "Back Panel" along normal blind 270
sketch "Switch Hole" plane through (0, 6, 0) normal (0, 1, 0) x (-1, 0, 0)
  line L0 (0, 0) -> (0, 500.8)
  line L1 (0, 500.8) -> (-270, 500.8)
  line L2 (-270, 500.8) -> (-270, 0)
  line L3 (-270, 0) -> (0, 0)
  line L4 (-234, 37) -> (-215, 37)
  line L5 (-215, 37) -> (-215, 24)
  line L6 (-215, 24) -> (-234, 24)
  line L7 (-234, 24) -> (-234, 37)
  dimension "d14" = 19
  dimension "d15" = 13
  dimension "d16" = 36
  dimension "d17" = 24
  constraint horizontal L4
  constraint vertical L5
  constraint horizontal L6
  constraint vertical L7
  measures "d14" distance of L5.end L6.end
  measures "d15" distance of L4.end L5.end
  measures "d16" distance of L2 L7
  measures "d17" distance of L3 L6
extrude "Extrude3" cut sketch "Switch Hole" against normal blind 6 contours L4 L5 L6 L7
sketch "Bottom Access Panel" plane through (0, 6, 0) normal (0, 1, 0) x (-1, 0, 0)
  line L0 (-215, 37) -> (-215, 24)
  line L1 (-215, 24) -> (-234, 24)
  line L2 (-234, 24) -> (-234, 37)
  line L3 (-234, 37) -> (-215, 37)
  line L4 (0, 0) -> (0, 500.8)
  line L5 (0, 500.8) -> (-270, 500.8)
  line L6 (-270, 500.8) -> (-270, 0)
  line L7 (-270, 0) -> (0, 0)
  line L8 (-205, 188) -> (-65, 188)
  line L9 (-65, 188) -> (-65, 48)
  line L10 (-65, 48) -> (-205, 48)
  line L11 (-205, 48) -> (-205, 188)
  dimension "d20" = 48
  dimension "d21" = 65
  dimension "d22" = 65
  dimension "d28" = 140
  dimension "d29" = 140
  dimension "d30" = 24
  dimension "d31" = 11
  dimension "d32" = 13
  dimension "d33" = 188
  constraint horizontal L8
  constraint vertical L9
  constraint horizontal L10
  constraint vertical L11
  measures "d20" distance of L7 L10
  measures "d21" distance of L6 L11
  measures "d22" distance of L4 L9
  measures "d28" distance of L8.end L9.end
  measures "d29" distance of L9.end L10.end
  measures "d30" distance of L1 L7
  measures "d31" distance of L3 L10
  measures "d32" distance of L1 L3
  measures "d33" distance of L7 L8
extrude "Extrude4" cut sketch "Bottom Access Panel" against normal blind 6 contours L8 L9 L10 L11
fillet "Fillet1" radius 8 4 edges at (65, 3, 188) (65, 3, 48) (205, 3, 48) (205, 3, 188)
sketch "Top Access Panel" plane through (0, 6, 0) normal (0, 1, 0) x (-1, 0, 0)
  line L0 (-65, 180) -> (-65, 56)
  arc A0 (-73, 48) -> (-65, 56) centre (-73, 56) ccw
  line L1 (-73, 48) -> (-197, 48)
  arc A1 (-205, 56) -> (-197, 48) centre (-197, 56) ccw
  line L2 (-205, 56) -> (-205, 180)
  arc A2 (-197, 188) -> (-205, 180) centre (-197, 180) ccw
  line L3 (-197, 188) -> (-73, 188)
  arc A3 (-65, 180) -> (-73, 188) centre (-73, 180) ccw
  line L4 (-215, 37) -> (-215, 24)
  line L5 (-215, 24) -> (-234, 24)
  line L6 (-234, 24) -> (-234, 37)
  line L7 (-234, 37) -> (-215, 37)
  line L8 (0, 0) -> (0, 500.8)
  line L9 (0, 500.8) -> (-270, 500.8)
  line L10 (-270, 500.8) -> (-270, 0)
  line L11 (-270, 0) -> (0, 0)
  line L12 (-195, 473.263) -> (-75, 473.263)
  line L13 (-75, 473.263) -> (-75, 383.263)
  line L14 (-75, 383.263) -> (-195, 383.263)
  line L15 (-195, 383.263) -> (-195, 473.263)
  line L16 (-180, 473.263) -> (-90, 473.263)
  line L17 (0, 503.263) -> (-270, 503.263)
  dimension "d34" = 120
  dimension "d35" = 140
  dimension "d36" = 75
  dimension "d37" = 75
  dimension "d38" = 65
  dimension "d39" = 65
  dimension "d45" = 90
  dimension "d49" = 30
  constraint horizontal L12
  constraint vertical L13
  constraint horizontal L14
  constraint vertical L15
  constraint coincident L12 L16.start
  measures "d34" distance of L13.end L14.end
  measures "d35" distance of L0 L2
  measures "d36" distance of L10 L15
  measures "d37" distance of L8 L13
  measures "d38" distance of L2 L10
  measures "d39" distance of L0 L8
  measures "d45" distance of L12.end L13.end
  measures "d49" distance of L16 L17
extrude "Extrude5" cut sketch "Top Access Panel" against normal blind 6 contours L12 L13 L14 L15 L16
fillet "Fillet2" radius 8 4 edges at (75, 3, 473.263) (195, 3, 473.263) (195, 3, 383.263) (75, 3, 383.263)
equation "MDFThickness = 6 mm"
equation "d16 = ( 18 * 2 ) * 1 mm"
equation "d17 = ( 12 * 2 ) * 1 mm"
equation "filletRadius = 8 mm"
equation "d27 = filletRadius"
equation "d36 = ( ( 270 - 120 ) / 2 ) * 1 mm"
equation "d54 = filletRadius"

design "Control Panel Support Right"
Autodesk Fusion 360 part; units mm, degrees
sketch "Control Panel Support" plane through (0, 0, 0) normal (1, 0, 0) x (0, 1, 0)
  line L0 (0, 0) -> (59, 0)
  line L1 (59, 0) -> (59, 43)
  line L2 (59, 43) -> (0, 43)
  line L3 (0, 43) -> (0, 0)
  dimension "d1" = 59
  dimension "d2" = 43
  constraint horizontal L0
  constraint vertical L1
  constraint horizontal L2
  constraint vertical L3
  constraint coincident L0.start L3.end
  measures "d1" distance of L0.start L0.end
  measures "d2" distance of L0.end L1.end
extrude "Extrude1" add sketch "Control Panel Support" along normal blind 12
equation "d1 = 65 mm - mdfThickness"
equation "pineThickness = 12 mm"
equation "d4 = pineThickness"
equation "mdfThickness = 6 mm"

design "Left Side Panel"
Autodesk Fusion 360 part; units mm, degrees
sketch "Side Panel" plane through (0, 0, 0) normal (1, 0, 0) x (0, 1, 0)
  line L0 (0, 0) -> (195, 0)
  line L1 (195, 0) -> (195, 520)
  line L2 (195, 520) -> (-0.3488, 600)
  line L3 (-0.3488, 600) -> (-0.3488, 510)
  line L4 (-0.3488, 510) -> (90, 473)
  line L5 (90, 473) -> (25, 345)
  line L6 (25, 345) -> (-65, 345)
  line L7 (-65, 345) -> (-65, 270)
  line L8 (-65, 270) -> (0, 270)
  line L9 (0, 270) -> (0, 0)
  dimension "d7" = 600
  dimension "d10" = 195
  dimension "d12" = 520
  dimension "d14" = 90
  dimension "d16" = 105
  dimension "d18" = 270
  dimension "d20" = 75
  dimension "d22" = 37
  dimension "d27" = 260
  dimension "d28" = 90
  dimension "d31" = 345
  constraint coincident L0.start L9.end
  constraint horizontal L0
  constraint perpendicular L0 L1
  constraint parallel L1 L3
  constraint parallel L2 L4
  constraint parallel L3 L7
  constraint perpendicular L7 L8
  constraint perpendicular L0 L9
  measures "d7" distance of L0 L2.end
  measures "d10" distance of L0.start L0.end
  measures "d12" distance of L0.end L1.end
  measures "d14" distance of L2.end L3.end
  measures "d16" distance of L1 L4.end
  measures "d18" distance of L8.end L0.start
  measures "d20" distance of L6.end L7.end
  measures "d22" distance of L3.end L4.end
  measures "d27" distance of L1 L7
  measures "d28" distance of L5.end L6.end
  measures "d31" distance of L0.start L5.end
extrude "Extrude1" add sketch "Side Panel" along normal blind 6
fillet "Fillet1" radius 8 10 edges at (3, -65, 345) (3, 25, 345) (3, 90, 473) (3, -0.3488, 510) (3, -0.3488, 600) (3, 195, 520) (3, -65, 270) (3, 0, 270) (3, 0, 0) (3, 195, 0)
sketch "Paint border" plane through (6, 0, 0) normal (1, 0, 0) x (0, 1, 0)
  arc A0 (187, 0) -> (195, 8) centre (187, 8) ccw
  line L0 (195, 8) -> (195, 514.6313)
  arc A1 (195, 514.6313) -> (190.0318, 522.0346) centre (187, 514.6313) ccw
  line L1 (190.0318, 522.0346) -> (10.683, 595.4822)
  arc A2 (10.683, 595.4822) -> (-0.3488, 588.079) centre (7.6512, 588.079) ccw
  line L2 (-0.3488, 588.079) -> (-0.3488, 515.3687)
  arc A3 (-0.3488, 515.3687) -> (4.6194, 507.9654) centre (7.6512, 515.3687) ccw
  line L3 (4.6194, 507.9654) -> (81.9699, 476.2885)
  arc A4 (86.0711, 465.263) -> (81.9699, 476.2885) centre (78.9381, 468.8853) ccw
  line L4 (86.0711, 465.263) -> (27.2231, 349.3778)
  arc A5 (20.0901, 345) -> (27.2231, 349.3778) centre (20.0901, 353) ccw
  line L5 (20.0901, 345) -> (-57, 345)
  arc A6 (-57, 345) -> (-65, 337) centre (-57, 337) ccw
  line L6 (-65, 337) -> (-65, 278)
  arc A7 (-65, 278) -> (-57, 270) centre (-57, 278) ccw
  line L7 (-57, 270) -> (-8, 270)
  arc A8 (0, 262) -> (-8, 270) centre (-8, 262) ccw
  line L8 (0, 262) -> (0, 8)
  arc A9 (0, 8) -> (8, 0) centre (8, 8) ccw
  line L9 (8, 0) -> (187, 0)
  line L10 (10, 6) -> (185, 6)
  line L11 (10, 6) -> (10, 280)
  line L12 (10, 280) -> (-55, 280)
  line L13 (-55, 280) -> (-55, 335)
  line L14 (-55, 335) -> (31.1374, 335)
  line L15 (9.6512, 516.7108) -> (103.8274, 478.1434)
  line L16 (31.1374, 335) -> (103.8274, 478.1434)
  line L17 (187.0159, 512.4636) -> (185, 6)
  line L18 (9.6512, 585.0987) -> (187.0159, 512.4636)
  line L19 (9.6512, 585.0987) -> (9.6512, 516.7108)
  dimension "d32" = 6
  dimension "d33" = 10
  dimension "d34" = 10
  dimension "d35" = 10
  dimension "d36" = 10
  dimension "d37" = 10
  dimension "d41" = 10
  dimension "d42" = 10
  dimension "d43" = 10
  dimension "d44" = 10
  constraint perpendicular L8 L10
  constraint perpendicular L10 L11
  constraint perpendicular L11 L12
  constraint perpendicular L12 L13
  constraint perpendicular L13 L14
  constraint parallel L3 L15
  constraint parallel L4 L16
  measures "d32" distance of L9 L10
  measures "d33" distance of L0 L10.end
  measures "d34" distance of L8 L10.start
  measures "d35" distance of L7 L11.end
  measures "d36" distance of L6 L12.end
  measures "d37" distance of L5 L13.end
  measures "d41" distance of L3 L15
  measures "d42" distance of L4 L16
  measures "d43" distance of L1 L18
  measures "d44" distance of L2 L19
extrude "Extrude2" cut sketch "Paint border" against normal blind 0.1
equation "MDFThickness = 6 mm"
equation "filletRadius = 8 mm"
equation "d3 = MDFThickness"
equation "d6 = filletRadius"
equation "d7 = totaHeight"
equation "totaHeight = 600 mm"
equation "baseWidth = 195 mm"
equation "d10 = baseWidth"
equation "backHight = 520 mm"
equation "d12 = backHight"
equation "namePanelHeight = 90 mm"
equation "d14 = namePanelHeight"
equation "neckWidth = 105 mm"
equation "d16 = neckWidth"
equation "bottomFrontHeight = 270 mm"
equation "d18 = bottomFrontHeight"
equation "controlPanelHeight = 75 mm"
equation "d20 = controlPanelHeight"
equation "namePanelFrontDipHeight = 37 mm"
equation "d22 = namePanelFrontDipHeight"
equation "controlPanelTopWidth = 90 mm"
equation "controlPanelTotalWidth = 260 mm"
equation "d27 = controlPanelTotalWidth"
equation "d28 = controlPanelTopWidth"
equation "d31 = bottomFrontHeight + controlPanelHeight"

design "Back Label"
Autodesk Fusion 360 part; units mm, degrees
sketch "Sticker" plane through (0, 0, 0) normal (0, 1, 0) x (1, 0, 0)
  line L0 (0, 0) -> (20, 0)
  line L1 (20, 0) -> (20, -12)
  line L2 (20, -12) -> (0, -12)
  line L3 (0, -12) -> (0, 0)
  dimension "d1" = 12
  dimension "d2" = 20
  constraint horizontal L0
  constraint vertical L1
  constraint horizontal L2
  constraint vertical L3
  constraint coincident L0.start L3.end
  measures "d1" distance of L0.end L1.end
  measures "d2" distance of L0.start L0.end
extrude "Extrude1" add sketch "Sticker" along normal blind 0.01 makes body 1
sketch "Text" plane through (0, 0, 0) normal (0, -1, 0) x (1, 0, 0)
  line L0 (20, 12) -> (0, 12)
  line L1 (0, 12) -> (0, 0)
  line L2 (0, 0) -> (20, 0)
  line L3 (20, 0) -> (20, 12)
  line L4 (0, 0) -> (20, 0) construction
  line L5 (20, 0) -> (20, 12) construction
  line L6 (20, 12) -> (0, 12) construction
  line L7 (0, 12) -> (0, 0) construction
  dimension "d5" = 5
  text T0 "Back" font "Arial" height 5 align centre middle in box 20 x 12 at (0, 0) x (1, 0) y (0, 1) spacing 1 kerned
  constraint coincident L2.end
  constraint coincident L0.end
extrude "Extrude2" add sketch "Text" along normal blind 0.01 separate body text T0 makes body 2 at (14.6982, 0, 5.8829) makes body 3 at (11.2962, 0, 4.2151) makes body 4 at (9.8356, 0, 4.5282) makes body 5 at (2.7257, 0, 5.9363)

design "Neodymium Disc Magnet"
Autodesk Fusion 360 part; units mm, degrees
sketch "Diameter" plane through (0, 0, 0) normal (0, 0, 1) x (1, 0, 0)
  circle A0 centre (0, 0) radius 2.5
  dimension "d1" = 5
  constraint coincident A0.centre origin
  measures "d1" diameter of A0
extrude "Extrude1" add sketch "Diameter" along normal blind 1.5
fillet "Fillet1" radius 0.05 2 edges at (-2.3308, -0.904, 1.5) (-2.3308, -0.904, 0)

design "Control Panel Support Left"
Autodesk Fusion 360 part; units mm, degrees
sketch "Control Panel Support" plane through (0, 0, 0) normal (1, 0, 0) x (0, 1, 0)
  line L0 (0, 0) -> (59, 0)
  line L1 (59, 0) -> (59, 43)
  line L2 (59, 43) -> (0, 43)
  line L3 (0, 43) -> (0, 0)
  dimension "d1" = 59
  dimension "d2" = 43
  constraint horizontal L0
  constraint vertical L1
  constraint horizontal L2
  constraint vertical L3
  constraint coincident L0.start L3.end
  measures "d1" distance of L0.start L0.end
  measures "d2" distance of L0.end L1.end
extrude "Extrude1" add sketch "Control Panel Support" along normal blind 12
equation "d1 = 65 mm - mdfThickness"
equation "pineThickness = 12 mm"
equation "d4 = pineThickness"
equation "mdfThickness = 6 mm"

design "Arcade Buttons Conduit"
Autodesk Fusion 360 part; units mm, degrees
sketch "16 mm x 16 mm conduit piping shape" plane through (0, 0, 0) normal (1, 0, 0) x (0, 1, 0)
  line L0 (0, 0) -> (16, 0)
  line L1 (16, 0) -> (16, 10)
  line L2 (16, 10) -> (14, 13.9)
  line L3 (14, 13.9) -> (13.1102, 13.4437)
  line L4 (13.1102, 13.4437) -> (15, 9.7585)
  line L5 (15, 9.7585) -> (15, 1)
  line L6 (15, 1) -> (1, 1)
  line L7 (1, 1) -> (1, 9.7585)
  line L8 (1, 9.7585) -> (2.8898, 13.4437)
  line L9 (2.8898, 13.4437) -> (2, 13.9)
  line L10 (2, 13.9) -> (0, 10)
  line L11 (0, 10) -> (0, 0)
  line L12 (0, 16) -> (16, 16)
  line L13 (0, 16) -> (0, 12)
  line L14 (0, 12) -> (1, 12)
  line L15 (1, 12) -> (1, 15)
  line L16 (1, 15) -> (15, 15)
  line L17 (15, 15) -> (15, 12)
  line L18 (15, 12) -> (16, 12)
  line L19 (16, 12) -> (16, 16)
  dimension "d1" = 1
  dimension "d2" = 16
  dimension "d3" = 1
  dimension "d4" = 1
  dimension "d7" = 10
  dimension "d8" = 10
  dimension "d9" = 16
  dimension "d10" = 1
  dimension "d11" = 1
  dimension "d12" = 1
  dimension "d13" = 4
  dimension "d14" = 4
  dimension "d15" = 16
  dimension "d16" = 2
  dimension "d17" = 2
  dimension "d18" = 1
  dimension "d19" = 1
  constraint coincident L0.start L11.end
  constraint horizontal L0
  constraint perpendicular L0 L1
  constraint perpendicular L2 L3
  constraint parallel L1 L5
  constraint perpendicular L5 L6
  constraint perpendicular L6 L7
  constraint perpendicular L0 L11
  constraint horizontal L12
  constraint perpendicular L12 L13
  constraint perpendicular L13 L14
  constraint perpendicular L14 L15
  constraint perpendicular L15 L16
  constraint perpendicular L16 L17
  constraint perpendicular L17 L18
  constraint perpendicular L12 L19
  constraint parallel L8 L10
  constraint parallel L2 L4
  constraint perpendicular L9 L10
  measures "d1" distance of L0 L6
  measures "d2" distance of L1 L11
  measures "d3" distance of L7 L11
  measures "d4" distance of L1 L5
  measures "d7" distance of L0.end L1.end
  measures "d8" distance of L10.end L0.start
  measures "d9" distance of L0 L12
  measures "d10" distance of L12 L16
  measures "d11" distance of L17 L19
  measures "d12" distance of L13 L15
  measures "d13" distance of L12.end L18.end
  measures "d14" distance of L12.start L13.end
  measures "d15" distance of L12.start L12.end
  measures "d16" distance of L1.end L2.end
  measures "d17" distance of L9.end L10.end
  measures "d18" distance of L2.end L3.end
  measures "d19" distance of L8.end L9.end
extrude "Extrude1" add sketch "16 mm x 16 mm conduit piping shape" along normal blind 212 makes body 1 at (70.6667, 5.3333, 16) makes body 2 at (70.6667, 5.3333, 0)
fillet "Fillet1" radius 0.3 18 edges at (106, 0, 16) (106, 16, 16) (106, 16, 12) (106, 0, 12) (106, 1, 12) (106, 15, 12) (106, 1, 15) (106, 15, 15) (106, 0, 10) (106, 16, 10) (106, 14, 13.9) (106, 13.1102, 13.4437) (106, 2, 13.9) (106, 2.8898, 13.4437) (106, 15, 1) (106, 1, 1) (106, 1, 9.7585) (106, 15, 9.7585) on bodies 1 2
sketch "Sketch2" plane through (0, 0, 0) normal (0, 1, 0) x (1, 0, 0)
  line L0 (13, -1) -> (25, -1)
  line L1 (25, -1) -> (25, -13.9551)
  line L2 (25, -13.9551) -> (13, -13.9551)
  line L3 (13, -13.9551) -> (13, -1)
  line L4 (63, -1) -> (75, -1)
  line L5 (75, -1) -> (75, -13.8889)
  line L6 (75, -13.8889) -> (63, -13.8889)
  line L7 (63, -13.8889) -> (63, -1)
  line L8 (113, -1) -> (125, -1)
  line L9 (125, -1) -> (125, -13.8172)
  line L10 (125, -13.8172) -> (113, -13.8172)
  line L11 (113, -13.8172) -> (113, -1)
  line L12 (0, -9.9276) -> (0, 0)
  line L13 (0, 0) -> (212, 0)
  dimension "d24" = 12
  dimension "d25" = 12
  dimension "d26" = 12
  dimension "d27" = 13
  dimension "d28" = 38
  dimension "d29" = 38
  dimension "d30" = 1
  dimension "d31" = 1
  dimension "d32" = 1
  constraint horizontal L0
  constraint vertical L1
  constraint horizontal L2
  constraint vertical L3
  constraint horizontal L4
  constraint vertical L5
  constraint horizontal L6
  constraint vertical L7
  constraint horizontal L8
  constraint vertical L9
  constraint horizontal L10
  constraint vertical L11
  measures "d24" distance of L0.start L0.end
  measures "d25" distance of L4.start L4.end
  measures "d26" distance of L8.start L8.end
  measures "d27" distance of L3 L12
  measures "d28" distance of L1 L7
  measures "d29" distance of L5 L11
  measures "d30" distance of L0 L13
  measures "d31" distance of L4 L13
  measures "d32" distance of L8 L13
extrude "Extrude2" cut sketch "Sketch2" along normal blind 3 bodies 2
equation "d1 = conduitThickness"
equation "d2 = conduitWidth"
equation "d3 = conduitThickness"
equation "d4 = conduitThickness"
equation "conduitThickness = 1 mm"
equation "conduitWidth = 16 mm"
equation "d9 = conduitWidth"
equation "d10 = conduitThickness"
equation "d11 = conduitThickness"
equation "d12 = conduitThickness"

design "Control Panel Top"
Autodesk Fusion 360 part; units mm, degrees
sketch "Control Panel Top" plane through (0, 0, 0) normal (0, 0, 1) x (1, 0, 0)
  line L0 (0, 0) -> (270, 0)
  line L1 (270, 0) -> (270, 86.085)
  line L2 (270, 86.085) -> (0, 86.085)
  line L3 (0, 86.085) -> (0, 0)
  dimension "d6" = 270
  dimension "d7" = 86.085
  constraint horizontal L0
  constraint vertical L1
  constraint horizontal L2
  constraint vertical L3
  constraint coincident L0.start L3.end
  measures "d6" distance of L0.start L0.end
  measures "d7" distance of L0.end L1.end
extrude "Extrude1" add sketch "Control Panel Top" along normal blind 6